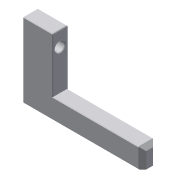
# Autodesk Inventor part: index finger
Saved by Autodesk Inventor 2022 Beta2 (Build 260130000, 130) ContinuousBuild 0
## iProperties
Shininess: 21.0
Length Units: 11272
Angle Units: 11279
Time Units: 11290
Mass Units: 11286
Length Display Precision: 3
Angle Display Precision: 2
Created: 2001-07-19
Part Number: index finger
Document SubType Name: Modeling
Designer: smithga
Density: 1 g/cm^3
Material: Generic
Appearance: Plastic-White
Density: 0.0
Volumn: 0.0
Area: 0.0
PropertySet Name: Model Information
Control State: 0
Master: False
Checked Out: False
Author: smithga
Autodesk Inventor part; units mm, degrees
ref_plane "YZ Plane" through (0, 0, 0) normal (1, 0, 0) x (0, 1, 0)
ref_plane "XZ Plane" through (0, 0, 0) normal (0, 1, 0) x (-1, 0, 0)
ref_plane "XY Plane" through (0, 0, 0) normal (0, 0, 1) x (1, 0, 0)
sketch "Sketch1" plane through (0, 0, 0) normal (0, 0, 1) x (1, 0, 0)
  line L0 (-57.15, 34.925) -> (-76.2, 34.925)
  line L1 (-76.2, 34.925) -> (-76.2, -12.7)
  line L2 (-76.2, -12.7) -> (0, -12.7)
  line L3 (0, -12.7) -> (0, 0)
  line L4 (0, 0) -> (-57.15, 0)
  line L5 (-57.15, 0) -> (-57.15, 34.925)
  constraints: 12 end point, 4 parallel, 1 horizontal, 1 perpendicular
extrude "Extrusion1" add sketch "Sketch1" along normal blind 9.525
chamfer "Chamfer4" distance 2.54 angle 45 3 edges at (0, 0, 4.7625) (0, -6.35, 9.525) (0, -6.35, 0)
chamfer "Chamfer2" distance 0.381 angle 45 12 edges at (-76.2, 34.925, 4.7625) (-57.15, 34.925, 4.7625) (-57.15, 17.4625, 9.525) (-66.675, 34.925, 9.525) (-66.675, 34.925, 0) (-76.2, 11.1125, 9.525) (-76.2, 11.1125, 0) (-29.845, 0, 9.525) (-29.845, 0, 0) (-39.37, -12.7, 9.525) (-76.2, -12.7, 4.7625) (-39.37, -12.7, 0)
sketch "Sketch2" plane through (-76.2, -12.319, 0.381) normal (-1, 0, 0) x (0, 0, 1)
  circle A0 centre (4.3815, 37.719) radius 3.175
  line L0 (-0.381, 46.863) -> (-0.381, 0) projected
  line L1 (8.763, 47.244) -> (0, 47.244) projected
  dimension "d6" = 4.7625
  dimension "d7" = 9.525
  constraints: 1 centre point
  measures "d6" distance from line of A0.centre L0
  measures "d7" distance from line of A0.centre L1
extrude "Extrusion2" cut sketch "Sketch2" against normal through all
chamfer "Chamfer3" distance 0.381 angle 45 2 edges at (-57.15, 25.4, 1.5875) (-76.2, 25.4, 1.5875)
body "Solid1"
